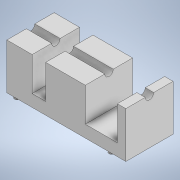
# Autodesk Inventor part: support_2
Saved by Autodesk Inventor 2021 (Build 250183000, 183)
## iProperties
Created: 2021-04-13
Part Number: support_2
Material: Generic
Document SubType Name: Modeling
Designer: Jawal
Density: 1 g/cm^3
Appearance: Default
Author: Jawal
Autodesk Inventor part; units mm, degrees
ref_plane "YZ Plane" through (0, 0, 0) normal (1, 0, 0) x (0, 1, 0)
ref_plane "XZ Plane" through (0, 0, 0) normal (0, 1, 0) x (-1, 0, 0)
ref_plane "XY Plane" through (0, 0, 0) normal (0, 0, 1) x (1, 0, 0)
sketch "Sketch7" plane through (0, 0, 0) normal (0, 1, 0) x (-1, 0, 0)
  line L0 (35, 14.012) -> (-35.5, 14.012)
  line L1 (-35.5, 14.012) -> (-35.5, -14.012)
  line L2 (-35.5, -14.012) -> (35, -14.012)
  line L3 (35, -14.012) -> (35, 14.012)
  point P0 (0, 0)
  dimension "d32" = 70.5
  dimension "d34" = 28.024
  dimension "d35" = 14.012
  constraints: 8 end point, 2 parallel, 1 horizontal, 1 perpendicular
  measures "d32" distance of L1.end L2.end
  measures "d34" distance of L2.end L0.start
  measures "d35" distance from line of L2 point (0, 0)
extrude "Extrusion3" add sketch "Sketch7" along normal blind 27.147
sketch "Sketch8" plane through (-35, 0, 14.012) normal (0, 0, 1) x (1, 0, 0)
  line L0 (70.5, 27.147) -> (0, 27.147) projected
  line L1 (15, 27.147) -> (23, 27.147)
  line L2 (23, 27.147) -> (23, 7.147)
  line L3 (23, 7.147) -> (15, 7.147)
  line L4 (15, 7.147) -> (15, 27.147)
  line L5 (0, 0) -> (0, 27.147) projected
  line L6 (46.5, 27.147) -> (65.5, 27.147)
  line L7 (65.5, 27.147) -> (65.5, 7.147)
  line L8 (65.5, 7.147) -> (46.5, 7.147)
  line L9 (46.5, 7.147) -> (46.5, 27.147)
  line L10 (70.5, 0) -> (70.5, 27.147) projected
  point P0 (35, 0)
  point P1 (23, 27.147)
  dimension "d39" = 20
  dimension "d40" = 15
  dimension "d41" = 8
  dimension "d42" = 46.5
  dimension "d44" = 5
  constraints: 16 end point, 4 parallel, 2 horizontal, 2 perpendicular, 2 point on line
  measures "d39" distance of L1.end L2.end
  measures "d40" distance between parallel lines of L5 L4
  measures "d41" distance of L2.end L3.end
  measures "d42" distance between parallel lines of L9 L5
  measures "d44" distance between parallel lines of L7 L10
extrude "Extrusion4" cut sketch "Sketch8" against normal through all
sketch "Sketch9" plane through (-35, 0, -14.012) normal (-1, 0, 0) x (0, 0, 1)
  line L0 (0, 27.147) -> (28.024, 27.147) projected
  arc A0 (11.512, 27.147) -> (16.512, 27.147) centre (14.012, 27.147) ccw
  point P0 (14.012, 0)
  dimension "d47" = 5
  constraints: 2 point on circle, 2 point on line, 1 centre point, 1 midpoint
  measures "d47" diameter of A0
extrude "Extrusion5" cut sketch "Sketch9" against normal through all
sketch "Sketch10" plane through (0, 0, 0) normal (0, -1, 0) x (1, 0, 0)
  circle A0 centre (-32.5, 10.512) radius 1.5
  line L0 (-35, -14.012) -> (-35, 14.012) projected
  circle A1 centre (23.5, 10.512) radius 1.5
  line L1 (35.5, 14.012) -> (35.5, -14.012) projected
  line L2 (-35, 14.012) -> (35.5, 14.012) projected
  point P0 (0, 0)
  dimension "d50" = 3
  dimension "d51" = 2.5
  dimension "d52" = 3
  dimension "d56" = 56
  dimension "d57" = 3.5
  dimension "d58" = 3.5
  constraints: 2 centre point
  measures "d50" diameter of A0
  measures "d51" distance from line of L0 A0.centre
  measures "d52" diameter of A1
  measures "d56" distance of A1.centre A0.centre
  measures "d57" distance from line of L2 A0.centre
  measures "d58" distance from line of L2 A1.centre
extrude "Extrusion6" add sketch "Sketch10" along normal blind 3
equation "\"d35\" = 0.5 * d34"
body "Solid2"
